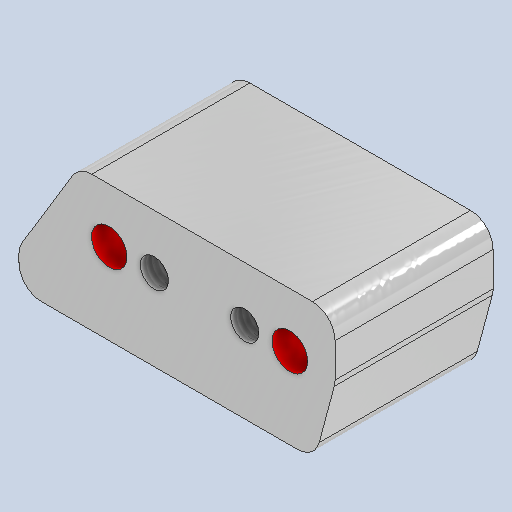
# Autodesk Inventor part: BRACE,CHAIN,#25,ELEVATOR
Saved by Autodesk Inventor 2025.2 (Build 292293000, 293)
## iProperties
ILogicPurgeVersion: 0.0.0.0
OnSaveVersion: 3.4.3.0
OnSaveAssembly: COREAutomationManager
Created: 2025-01-28
Part Number: BRACE,CHAIN,#25,ELEVATOR
Material: Aluminum 7075
Document SubType Name: Modeling
Designer: Jthib
Density: 2.81 g/cm^3
Appearance: Machined - Aluminum
Mfg Approved By: John.Thibert
ModelCat: Uncategorized
MaterialName: Aluminum 7075
CN_MASS: 0
Author: Jthib
Autodesk Inventor part; units mm, degrees
ref_plane "YZ Plane" through (0, 0, 0) normal (1, 0, 0) x (0, 1, 0)
ref_plane "XZ Plane" through (0, 0, 0) normal (0, 1, 0) x (-1, 0, 0)
ref_plane "XY Plane" through (0, 0, 0) normal (0, 0, 1) x (1, 0, 0)
sketch "Sketch1" plane through (0, 0, 0) normal (0, 0, 1) x (1, 0, 0)
  line L0 (19.05, 7.62) -> (-25.4, 7.62)
  line L1 (-25.4, 7.62) -> (-25.4, -11.43)
  line L2 (-25.4, -11.43) -> (19.05, -11.43)
  line L3 (19.05, -11.43) -> (19.05, 7.62)
  line L4 (19.05, 7.62) -> (-25.4, -11.43) construction
  line L5 (-25.4, 7.62) -> (19.05, -11.43) construction
  line L6 (0, 11.43) -> (0, -15.24) construction
  line L7 (-34.29, 0) -> (27.94, 0) construction
  point P0 (-3.175, -1.905)
  dimension "d0" = 19.05
  dimension "d1" = 44.45
  dimension "d56" = 25.4
  dimension "d93" = 11.43
  constraints: 12 end point, 2 parallel, 1 horizontal, 1 midpoint, 1 perpendicular
  measures "d0" distance of L0.end L1.end
  measures "d1" distance of L1.end L2.end
  measures "d56" distance between parallel lines of L6 L1
  measures "d93" distance between parallel lines of L7 L2
extrude "Extrusion1" add sketch "Sketch1" along normal mid plane 22.225
sketch "Sketch3" plane through (0, 0, 11.1125) normal (0, 0, 1) x (1, 0, 0)
  line L0 (-12.7, 0) -> (12.7, 0) construction
  point P0 (0, 0)
  point P1 (0, 0)
  dimension "d35" = 25.4
  constraints: 3 coincident, 2 end point, 1 horizontal, 1 midpoint
  measures "d35" distance of L0.start L0.end
hole "Hole1" at (-12.7, 0, 11.1125) at (12.7, 0, 11.1125) direction (0, 0, -1) diameter 5.0038 end through all clearance for "H7 - STANDARD FIT" size "5" standard "CL-DOWEL-MET"
sketch "Sketch4" plane through (0, 0, 11.1125) normal (0, 0, 1) x (1, 0, 0)
  line L0 (-6.35, 0) -> (6.35, 0) construction
  point P0 (0, 0)
  point P1 (0, 0)
  dimension "d43" = 12.7
  constraints: 3 coincident, 2 end point, 1 horizontal, 1 midpoint
  measures "d43" distance of L0.start L0.end
hole "Hole2" at (-6.35, 0, 11.1125) at (6.35, 0, 11.1125) direction (0, 0, -1) diameter 3.9624 end through all thread size "10-32 UNF" class "2B" standard "ANSI Unified Screw Threads"
sketch "Sketch6" plane through (-25.4, -11.43, 11.1125) normal (0, -1, 0) x (1, 0, 0)
  line L0 (25.4, -11.1125) -> (6.35, -11.1125) construction
  point P0 (12.7, -11.1125)
  point P1 (12.7, -11.1125)
  point P2 (19.05, -11.1125)
  point P3 (19.05, -11.1125)
  point P4 (25.4, -11.1125)
  point P5 (25.4, -11.1125)
  point P6 (31.75, -11.1125)
  point P7 (31.75, -11.1125)
  point P8 (25.4, -11.1125)
  dimension "d83" = 19.05
  dimension "d84" = 6.35
  constraints: 6 coincident, 3 end point, 2 horizontal, 8 other
  measures "d83" distance of L0.start L0.end
  measures "d84" distance of L0.end point (12.7, -11.113)
hole "Hole4" at (-19.05, -11.43, 0) at (-12.7, -11.43, 0) at (-6.35, -11.43, 0) at (0, -11.43, 0) at (6.35, -11.43, 0) direction (0, 1, 0) diameter 2.459 depth 8.7884 tip angle 118 thread size "M3x0.5" class "6H" standard "ANSI Metric M Profile"
chamfer "Chamfer2" distance 10.668 angle 15 1 edges at (19.05, -11.43, 0) measured on face at (19.05, -10.93, 0)
chamfer "Chamfer3" distance 13.97 angle 31.215 1 edges at (-25.4, 7.62, 0) measured on face at (-25.4, 7.12, 0)
fillet "Fillet1" radius 3.175 6 edges at (16.1915, -11.43, 0) (-25.4, -11.43, 0) (-25.4, -6.35, 0) (-16.9346, 7.62, 0) (19.05, 7.62, 0) (19.05, -0.762, 0)
body "Solid1"
